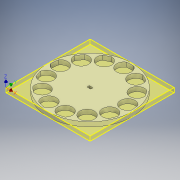
# Autodesk Inventor part: レスキューキット投下機構
Saved by Autodesk Inventor 2018 (Build 220112000, 112)
## iProperties
Created: 2018-08-16
Part Number: レスキューキット投下機構
Material: 一般
Document SubType Name: Modeling
Designer: shun2
Density: 1 g/cm^3
Appearance: 既定
Author: shun2
Autodesk Inventor part; units mm, degrees
ref_plane "YZ Plane" through (0, 0, 0) normal (1, 0, 0) x (0, 1, 0)
ref_plane "XZ Plane" through (0, 0, 0) normal (0, 1, 0) x (-1, 0, 0)
ref_plane "XY Plane" through (0, 0, 0) normal (0, 0, 1) x (1, 0, 0)
sketch "スケッチ1" plane through (0, 0, 0) normal (0, 0, 1) x (1, 0, 0)
  circle A0 centre (65, 55.362) radius 52
  circle A1 centre (65, 55.362) radius 52
  arc A2 (60.5059, 105.1596) -> (69.4941, 105.1596) centre (65, 97.362) ccw
  arc A3 (37.8785, 97.367) -> (45.8372, 101.5441) centre (45.4816, 92.5511) ccw
  arc A4 (21.4644, 79.9516) -> (26.5703, 87.3488) centre (30.4347, 79.2207) ccw
  arc A5 (15.0238, 56.903) -> (16.1072, 65.8258) centre (23.3062, 60.4245) ccw
  arc A6 (20.0321, 33.5014) -> (16.8448, 41.9056) centre (25.7293, 40.4686) ccw
  arc A7 (35.342, 15.1078) -> (28.6142, 21.0681) centre (37.1488, 23.9245) ccw
  arc A8 (57.4462, 5.9359) -> (48.7191, 8.0869) centre (54.9487, 14.5824) ccw
  arc A9 (81.2809, 8.0869) -> (72.5538, 5.9359) centre (75.0513, 14.5824) ccw
  arc A10 (101.3858, 21.0681) -> (94.658, 15.1078) centre (92.8512, 23.9245) ccw
  arc A11 (113.1552, 41.9056) -> (109.9679, 33.5014) centre (104.2707, 40.4686) ccw
  arc A12 (113.8928, 65.8258) -> (114.9762, 56.903) centre (106.6938, 60.4245) ccw
  arc A13 (103.4297, 87.3488) -> (108.5356, 79.9516) centre (99.5653, 79.2207) ccw
  arc A14 (84.1628, 101.5441) -> (92.1215, 97.367) centre (84.5184, 92.5511) ccw
  arc A15 (45.8372, 101.5441) -> (37.8785, 97.367) centre (65, 55.362) ccw
  arc A16 (69.4941, 105.1596) -> (60.5059, 105.1596) centre (65, 55.362) ccw
  arc A17 (92.1215, 97.367) -> (84.1628, 101.5441) centre (65, 55.362) ccw
  arc A18 (108.5356, 79.9516) -> (103.4297, 87.3488) centre (65, 55.362) ccw
  arc A19 (114.9762, 56.903) -> (113.8928, 65.8258) centre (65, 55.362) ccw
  arc A20 (109.9679, 33.5014) -> (113.1552, 41.9056) centre (65, 55.362) ccw
  arc A21 (94.658, 15.1078) -> (101.3858, 21.0681) centre (65, 55.362) ccw
  arc A22 (72.5538, 5.9359) -> (81.2809, 8.0869) centre (65, 55.362) ccw
  arc A23 (48.7191, 8.0869) -> (57.4462, 5.9359) centre (65, 55.362) ccw
  arc A24 (28.6142, 21.0681) -> (35.342, 15.1078) centre (65, 55.362) ccw
  arc A25 (16.8448, 41.9056) -> (20.0321, 33.5014) centre (65, 55.362) ccw
  arc A26 (26.5703, 87.3488) -> (21.4644, 79.9516) centre (65, 55.362) ccw
  arc A27 (16.1072, 65.8258) -> (15.0238, 56.903) centre (65, 55.362) ccw
  line L0 (63, 56.862) -> (67, 56.862)
  line L1 (67, 53.862) -> (63, 53.862)
  arc A28 (67, 53.862) -> (67, 56.862) centre (65, 55.362) ccw
  arc A29 (63, 56.862) -> (63, 53.862) centre (65, 55.362) ccw
  point P0 (0, 0)
  constraints: 56 point on circle, 30 centre point, 4 end point, 1 coincident, 1 horizontal, 1 parallel
extrude "押し出し1" add sketch "スケッチ1" along normal blind 5.5
